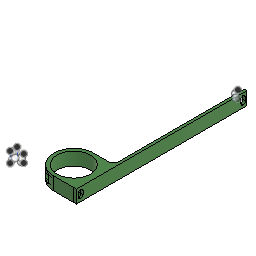
Eurohole v1 (Autodesk Fusion 360 design; units mm, degrees)
Autodesk Fusion 360 part; units mm, degrees
sketch "eurohole" plane through (0, 0, 0) normal (0, 0, 1) x (1, 0, 0)
  line L0 (148.7056, -33.4118) -> (148.7056, -127.9153)
  spline S0 degree 3 poles (148.7056, -127.9153) (148.7056, -130.1262) (146.9133, -131.9185) (144.7024, -131.9185) knots 1 1 1 1 2 2 2 2
  line L1 (144.7024, -131.9185) -> (133.7056, -131.9185)
  spline S1 degree 3 poles (133.7056, -131.9185) (125.4213, -131.9185) (118.7056, -138.6342) (118.7056, -146.9185) knots 3 3 3 3 4 4 4 4
  line L2 (118.7056, -146.9185) -> (118.7056, -146.9185)
  spline S2 degree 3 poles (118.7056, -146.9185) (118.7056, -155.2028) (125.4213, -161.9185) (133.7056, -161.9185) knots 5 5 5 5 6 6 6 6
  line L3 (133.7056, -161.9185) -> (148.7056, -161.9185)
  line L4 (148.7056, -161.9185) -> (148.7056, -161.9118)
  line L5 (148.7056, -161.9118) -> (150.7056, -161.9118)
  line L6 (150.7056, -161.9118) -> (150.7056, -33.4118)
  line L7 (150.7056, -33.4118) -> (148.7056, -33.4118)
  spline S3 degree 3 poles (133.7056, -159.4185) (126.802, -159.4185) (121.2056, -153.822) (121.2056, -146.9185) (121.2056, -140.0149) (126.802, -134.4185) (133.7056, -134.4185) (140.6092, -134.4185) (146.2056, -140.0149) (146.2056, -146.9185) (146.2056, -153.822) (140.6092, -159.4185) (133.7056, -159.4185) knots 0 0 0 0 1 1 1 2 2 2 3 3 3 4 4 4 4
extrude "Extrude1" add sketch "eurohole" along normal blind 9.8
move_body "Move1" bodies 1 to x (1, 0, 0) y (0, 1, 0) z (0, 0, 1) at (0, 33, 0)
move_body "Move2" bodies 1 to x (1, 0, 0) y (0, 1, 0) z (0, 0, 1) at (0, 0.5, 0)
move_body "Move3" bodies 1 to x (1, 0, 0) y (0, 1, 0) z (0, 0, 1) at (0, -0.09, 0)
sketch "Sketch2" plane through (0, 0, 0) normal (1, 0, 0) x (0, 1, 0)
  line L0 (-2.6319, 8, 145) -> (-2.9, 8, 145)
  line L1 (-4.5, 6.4, 145) -> (-4.5, 3.6, 145)
  line L2 (-2.9, 2, 145) -> (-2.6319, 2, 145)
  line L3 (-1.0319, 3.6, 145) -> (-1.0319, 6.4, 145)
  arc A0 through (-1.0319, 6.4, 145) (-1.5005, 7.5314, 145) (-2.6319, 8, 145)
  arc A1 through (-2.9, 8, 145) (-4.0314, 7.5314, 145) (-4.5, 6.4, 145)
  arc A2 through (-2.6319, 2, 145) (-1.5005, 2.4686, 145) (-1.0319, 3.6, 145)
  arc A3 through (-4.5, 3.6, 145) (-4.0314, 2.4686, 145) (-2.9, 2, 145)
  line L4 (-125.4, 2, 106) -> (-125.1319, 2, 106)
  arc A4 through (-127, 3.6, 106) (-126.5314, 2.4686, 106) (-125.4, 2, 106)
  arc A5 through (-123.5319, 6.4, 106) (-124.0005, 7.5314, 106) (-125.1319, 8, 106)
  arc A6 through (-125.4, 8, 106) (-126.5314, 7.5314, 106) (-127, 6.4, 106)
  arc A7 through (-125.1319, 2, 106) (-124.0005, 2.4686, 106) (-123.5319, 3.6, 106)
  line L5 (-125.1319, 8, 106) -> (-125.4, 8, 106)
  line L6 (-127, 6.4, 106) -> (-127, 3.6, 106)
  line L7 (-123.5319, 3.6, 106) -> (-123.5319, 6.4, 106)
  line L8 (-126.2767, 8.9878, 100) -> (-124.0267, 8.9878, 100)
  line L9 (-122.5267, 7.4878, 100) -> (-122.5267, 2.4878, 100)
  line L10 (-124.0267, 0.9878, 100) -> (-126.2767, 0.9878, 100)
  line L11 (-127.7767, 2.4878, 100) -> (-127.7767, 7.4878, 100)
  arc A8 through (-122.5267, 7.4878, 100) (-122.9661, 8.5484, 100) (-124.0267, 8.9878, 100)
  arc A9 through (-126.2767, 8.9878, 100) (-127.3374, 8.5484, 100) (-127.7767, 7.4878, 100)
  arc A10 through (-127.7767, 2.4878, 100) (-127.3374, 1.4271, 100) (-126.2767, 0.9878, 100)
  arc A11 through (-124.0267, 0.9878, 100) (-122.9661, 1.4271, 100) (-122.5267, 2.4878, 100)
  point P0 (-1.0319, 8)
  point P1 (-1.0319, 2)
  point P2 (-123.5319, 2)
  point P3 (-123.5319, 8)
  point P4 (-127.7767, 8.9878)
  point P5 (-122.5267, 8.9878)
  point P6 (-127.7767, 0.9878)
extrude "Extrude2" cut sketch "Sketch2" along normal blind 11 contours L0 L1 L2 L3 A0 A1 A2 A3 in plane through (145, 0, 0) normal (1, 0, 0)
extrude "Extrude3" cut sketch "Sketch2" along normal blind 46 contours L4 A4 A5 A6 A7 L5 L6 L7 in plane through (106, 0, 0) normal (1, 0, 0)
extrude "Extrude4" cut sketch "Sketch2" along normal blind 49 contours L8 L9 L10 L11 A8 A9 A10 A11 in plane through (100, 0, 0) normal (1, 0, 0)
